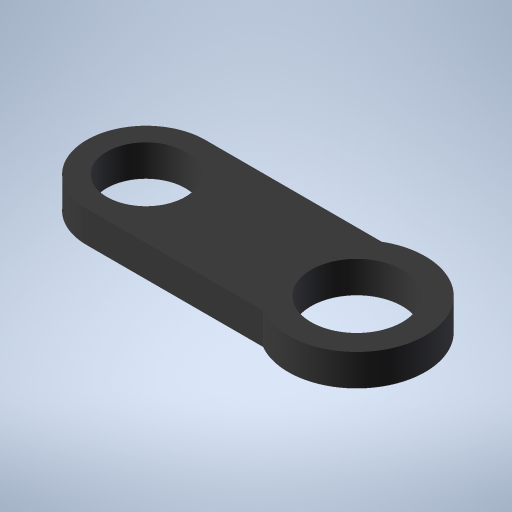
# Autodesk Inventor part: Connecting Rod
Saved by Autodesk Inventor 2023 (Build 270158000, 158)
## iProperties
Created: 2022-10-29
Part Number: Connecting Rod
Material: Generic
Document SubType Name: Modeling
Designer: tommy
Density: 1 g/cm^3
Appearance: Default
Author: tommy
Autodesk Inventor part; units mm, degrees
ref_plane "YZ Plane" through (0, 0, 0) normal (1, 0, 0) x (0, 1, 0)
ref_plane "XZ Plane" through (0, 0, 0) normal (0, 1, 0) x (-1, 0, 0)
ref_plane "XY Plane" through (0, 0, 0) normal (0, 0, 1) x (1, 0, 0)
sketch "Sketch1" plane through (0, 0, 0) normal (0, 1, 0) x (-1, 0, 0)
  arc A0 (-23.4767, 14.2875) -> (-23.4767, -14.2875) centre (-31.75, 0) ccw
  circle A1 centre (-31.75, 0) radius 10.9982
  circle A2 centre (19.05, 0) radius 9.4869
  arc A3 (19.05, -14.2875) -> (19.05, 14.2875) centre (19.05, 0) ccw
  line L0 (19.05, -14.2875) -> (-23.4767, -14.2875)
  line L1 (19.05, 14.2875) -> (-23.4767, 14.2875)
  point P0 (0, 0)
  point P1 (12.5046, 12.7)
  point P2 (-21.2006, -12.7)
  dimension "d11" = 18.9738
  dimension "d14" = 28.575
  constraints: 6 point on circle, 4 centre point, 4 end point, 2 coincident, 2 horizontal
  measures "d11" diameter of A2
  measures "d14" diameter of A3
extrude "Extrusion1" add sketch "Sketch1" along normal blind 7.62
body "Solid1"
